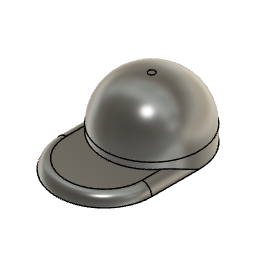
Cap (Autodesk Fusion 360 design; units mm, degrees)
Autodesk Fusion 360 part; units mm, degrees
sketch "Sketch2" plane through (0, 0, 0) normal (0, 0, 1) x (1, 0, 0)
  circle A0 centre (0, 0) radius 19.05
  dimension "d15" = 38.1
  constraint coincident A0.centre origin
  measures "d15" diameter of A0
extrude "Extrude1" add sketch "Sketch2" along normal blind 20.32
fillet "Fillet4" radius 17.78 1 edges at (-17.7608, -6.8888, 20.32)
sketch "Sketch5" plane through (0, 0, 0) normal (0, 0, -1) x (1, 0, 0)
  circle A0 centre (0, 19.05) radius 19.05
  line L0 (19.05, 0) -> (19.05, 19.05)
  line L1 (-19.05, 0) -> (-19.05, 19.05)
  circle A1 centre (0, 0) radius 19.05
  dimension "d22" = 38.1
  constraint coincident A0 L0.end
  constraint tangent A0 L0
  constraint vertical L0
  constraint coincident A0 L1.end
  constraint tangent A0 L1
  constraint vertical L1
  measures "d22" diameter of A0
extrude "Extrude4" add sketch "Sketch5" along normal blind 3.81
sketch "Sketch6" plane through (0, 0, -3.81) normal (0, 0, -1) x (1, 0, 0)
  line L0 (19.05, 0) -> (19.05, 19.05)
  arc A0 (19.05, 19.05) -> (-19.05, 19.05) centre (0, 19.05) ccw
  line L1 (-19.05, 19.05) -> (-19.05, 0)
  arc A1 (-19.05, 0) -> (19.05, 0) centre (0, 0) ccw
  circle A2 centre (0, 0) radius 12.7
  circle A3 centre (0, -12.7) radius 2.2098
  circle A4 centre (10.9985, 6.35) radius 2.2098
  circle A5 centre (-10.9985, 6.35) radius 2.2098
  dimension "d28" = 25.4
  dimension "d29" = 4.4196
  dimension "d31" = 360
  constraint concentric A1 A2
  constraint coincident A2 A3.centre
  measures "d28" diameter of A2
  measures "d29" diameter of A3
extrude "Extrude5" add sketch "Sketch6" along normal blind 5 contours A2 A4 | A2 A4 | A2 A3 | A2 A3 | A2 A5 | A2 A5
fillet "Fillet5" radius 3.81 3 edges at (19.05, -9.525, 0) (0, -38.1, 0) (-19.05, -9.525, 0)
